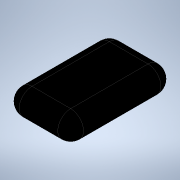
# Autodesk Inventor part: mapContainerPlaceholder
Saved by Autodesk Inventor 2020.3 (Build 243373000, 373)
## iProperties
Created: 2021-03-03
Part Number: mapContainerPlaceholder
Material: Generic
Document SubType Name: Modeling
Designer: con_c_000
Density: 1 g/cm^3
Appearance: Default
Author: con_c_000
Autodesk Inventor part; units mm, degrees
ref_plane "YZ Plane" through (0, 0, 0) normal (1, 0, 0) x (0, 1, 0)
ref_plane "XZ Plane" through (0, 0, 0) normal (0, 1, 0) x (-1, 0, 0)
ref_plane "XY Plane" through (0, 0, 0) normal (0, 0, 1) x (1, 0, 0)
sketch "Sketch1" plane through (0, 0, 0) normal (0, 0, 1) x (1, 0, 0)
  circle A0 centre (-5.4752, 0) radius 50.8
  circle A1 centre (146.9248, 0) radius 50.8
  line L0 (146.9248, 50.8) -> (-5.4752, 50.8)
  line L1 (-5.4752, -50.8) -> (146.9248, -50.8)
  point P0 (0, 0)
  dimension "d0" = 101.6
  dimension "d1" = 101.6
  dimension "d2" = 152.4
  constraints: 4 end point, 4 point on circle, 3 tangent, 2 centre point
  measures "d0" diameter of A0
  measures "d1" diameter of A1
  measures "d2" distance of A0.centre A1.centre
extrude "Extrusion1" add sketch "Sketch1" along normal blind 406.4
fillet "Fillet1" radius 50.8 4 edges at (-56.2752, 0, 406.4) (70.7248, -50.8, 406.4) (197.7248, 0, 406.4) (70.7248, 50.8, 406.4)
fillet "Fillet2" radius 50.8 4 edges at (-56.2752, 0, 0) (70.7248, -50.8, 0) (197.7248, 0, 0) (70.7248, 50.8, 0)
body "Solid1"
